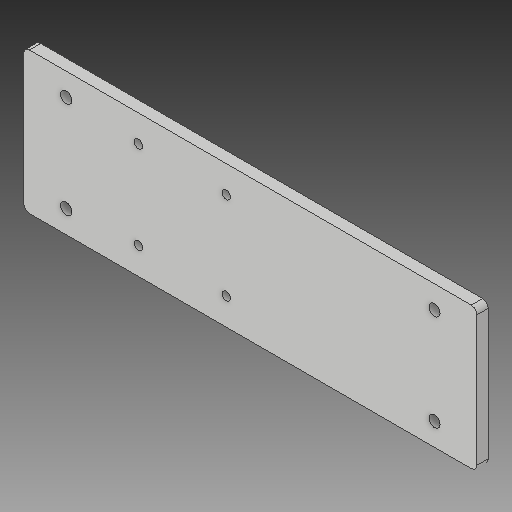
# Autodesk Inventor part: wiper motor holder
Saved by Autodesk Inventor 2019 (Build 230136000, 136)
## iProperties
Created: 2020-03-12
Part Number: wiper motor holder
Material: Generic
Document SubType Name: Modeling
Designer: Vijay
Density: 1 g/cm^3
Appearance: Default
Author: Vijay
Autodesk Inventor part; units mm, degrees
ref_plane "YZ Plane" through (0, 0, 0) normal (1, 0, 0) x (0, 1, 0)
ref_plane "XZ Plane" through (0, 0, 0) normal (0, 1, 0) x (-1, 0, 0)
ref_plane "XY Plane" through (0, 0, 0) normal (0, 0, 1) x (1, 0, 0)
sketch "Sketch1" plane through (0, 0, 0) normal (0, 0, 1) x (1, 0, 0)
  line L0 (139.9, -900) -> (139.9, 100) construction
  line L1 (-20.1001, -2.6886) -> (-20.0999, -902.6886) construction
  line L2 (139.9, -395.4885) -> (-20.1, -395.4885)
  line L3 (-20.1, -395.4885) -> (-20.1, -345.4885)
  line L4 (-20.1, -345.4885) -> (139.9, -345.4885)
  line L5 (139.9, -345.4885) -> (139.9, -395.4885)
  point P0 (0, 0)
  dimension "d0" = 50
  constraints: 10 end point, 2 parallel, 2 point on line, 1 horizontal, 1 perpendicular, 1 vertical, 2 other
  measures "d0" distance between parallel lines of L4 L2
extrude "Extrusion1" add sketch "Sketch1" along normal blind 4
fillet "Fillet1" radius 2 4 edges at (-20.1, -395.4885, 2) (-20.1, -345.4885, 2) (139.9, -395.4885, 2) (139.9, -345.4885, 2)
sketch "Sketch2" plane through (0, 0, 4) normal (0, 0, 1) x (1, 0, 0)
  line L0 (128.9999, 97.3115) -> (129.0001, -902.6885) construction
  line L1 (120.7999, 97.3115) -> (128.9999, 97.3115) construction
  line L2 (120.7999, 97.3115) -> (120.8001, -902.6885) construction
  line L3 (129.0001, -902.6885) -> (120.8001, -902.6885) construction
  line L4 (-1.0001, 97.3114) -> (-0.9999, -902.6886) construction
  line L5 (-9.2001, 97.3114) -> (-1.0001, 97.3114) construction
  line L6 (-9.2001, 97.3114) -> (-9.1999, -902.6886) construction
  line L7 (-0.9999, -902.6886) -> (-9.1999, -902.6886) construction
  line L8 (124.9001, -902.6885) -> (124.8999, 97.3115) construction
  line L9 (-5.1001, 97.3114) -> (-5.0999, -902.6886) construction
  circle A0 centre (51.3999, -385.9885) radius 1.5 construction
  circle A1 centre (20.3999, -385.9885) radius 1.5 construction
  circle A2 centre (20.3999, -354.9885) radius 1.5 construction
  circle A3 centre (51.3999, -354.9885) radius 1.5 construction
  circle A4 centre (124.9, -387.4885) radius 2
  circle A5 centre (124.9, -353.4885) radius 2
  circle A6 centre (51.3999, -385.9885) radius 1.5
  circle A7 centre (51.3999, -354.9885) radius 1.5
  circle A8 centre (20.3999, -354.9885) radius 1.5
  circle A9 centre (20.3999, -385.9885) radius 1.5
  circle A10 centre (-5.1, -387.4885) radius 2
  circle A11 centre (-5.1, -353.4885) radius 2
  line L10 (-18.1, -395.4885) -> (137.9, -395.4885) projected
  line L11 (137.9, -345.4885) -> (-18.1, -345.4885) projected
  point P0 (0, 0)
  dimension "d4" = 4
  dimension "d5" = 4
  dimension "d6" = 3
  dimension "d7" = 3
  dimension "d8" = 3
  dimension "d9" = 3
  dimension "d10" = 4
  dimension "d11" = 4
  dimension "d12" = 8
  dimension "d13" = 8
  dimension "d14" = 8
  dimension "d15" = 8
  constraints: 8 centre point, 4 coincident, 4 end point, 4 midpoint, 4 point on line
  measures "d4" diameter of A4
  measures "d5" diameter of A5
  measures "d6" diameter of A6
  measures "d7" diameter of A7
  measures "d8" diameter of A8
  measures "d9" diameter of A9
  measures "d10" diameter of A10
  measures "d11" diameter of A11
  measures "d12" distance from line of A4.centre L10
  measures "d13" distance from line of L11 A5.centre
  measures "d14" distance from line of A10.centre L10
  measures "d15" distance from line of L11 A11.centre
extrude "Extrusion2" cut sketch "Sketch2" against normal through all
body "Solid1"
